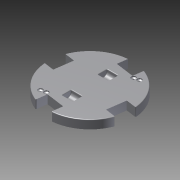
# Autodesk Inventor part: Outlet Cover [Top]
Saved by Autodesk Inventor 2012 (Build 160160000, 160)
## iProperties
Created: 2012-04-03
Part Number: Outlet Cover [Top]
Material: Default
Document SubType Name: Modeling
Designer: 21842
Density: 1 g/cm^3
Author: 21842
Autodesk Inventor part; units mm, degrees
ref_plane "YZ Plane" through (0, 0, 0) normal (1, 0, 0) x (0, 1, 0)
ref_plane "XZ Plane" through (0, 0, 0) normal (0, 1, 0) x (-1, 0, 0)
ref_plane "XY Plane" through (0, 0, 0) normal (0, 0, 1) x (1, 0, 0)
sketch "Sketch1" plane through (0, 0, 0) normal (0, 0, 1) x (1, 0, 0)
  circle A0 centre (-23.1688, -41.9) radius 3.5
  circle A1 centre (23.1688, 41.9) radius 3.5
  circle A2 centre (-30.3996, -43.4151) radius 3.5
  circle A3 centre (30.3996, 43.4151) radius 3.5
  circle A4 centre (-20.5794, 37.9797) radius 2.75
  circle A5 centre (20.5794, -37.9797) radius 2.75
  circle A6 centre (-30.3996, -43.4151) radius 1.6
  circle A7 centre (-23.1688, -41.9) radius 1.6
  circle A8 centre (23.1688, 41.9) radius 1.6
  circle A9 centre (30.3996, 43.4151) radius 1.6
  line L0 (-62.7781, -5.2832) -> (-47.4535, -7.4369)
  line L1 (-47.4535, -7.4369) -> (-43.6375, 19.715)
  line L2 (-43.6375, 19.715) -> (-59.0767, 21.8849)
  line L3 (5.2832, -62.7781) -> (7.4369, -47.4535)
  line L4 (7.4369, -47.4535) -> (-19.715, -43.6375)
  line L5 (-19.715, -43.6375) -> (-21.8849, -59.0767)
  line L6 (62.7781, 5.2832) -> (47.4535, 7.4369)
  line L7 (47.4535, 7.4369) -> (43.6375, -19.715)
  line L8 (43.6375, -19.715) -> (59.0767, -21.8849)
  line L9 (-5.2832, 62.7781) -> (-7.4369, 47.4535)
  line L10 (-7.4369, 47.4535) -> (19.715, 43.6375)
  line L11 (19.715, 43.6375) -> (21.8849, 59.0767)
  arc A10 (-5.2832, 62.7781) -> (-59.0767, 21.8849) centre (0, 0) ccw
  arc A11 (62.7781, 5.2832) -> (21.8849, 59.0767) centre (0, 0) ccw
  arc A12 (-62.7781, -5.2832) -> (-21.8849, -59.0767) centre (0, 0) ccw
  arc A13 (5.2832, -62.7781) -> (59.0767, -21.8849) centre (0, 0) ccw
  dimension "d0" = 3.2
  dimension "d1" = 3.2
  dimension "d2" = 3.2
  dimension "d3" = 3.2
  dimension "d8" = 360
  constraints: 24 end point, 14 centre point, 8 point on circle, 4 coincident, 29 other
  measures "d0" diameter of A6
  measures "d1" diameter of A7
  measures "d2" diameter of A8
  measures "d3" diameter of A9
extrude "Extrusion1" add sketch "Sketch1" along normal blind 12.7 contours A0 | A1 | A2 | A3 | A4 | A5 | L0 L1 L2 A10 L9 L10 L11 A11 L6 L7 L8 A13 L3 L4 L5 A12
extrude "Extrusion2" cut sketch "Sketch1" along normal blind 7 contours A4 | A5
hole "Hole1" at (30.3996, 43.4151, 12.7) direction (0, 0, -1) diameter 7 depth 1.5 tip angle 118
hole "Hole2" at (23.1688, 41.9, 12.7) direction (0, 0, -1) diameter 7 depth 1.5 tip angle 118
hole "Hole3" at (-23.1688, -41.9, 12.7) direction (0, 0, -1) diameter 7 depth 1.5 tip angle 118
hole "Hole4" at (-30.3996, -43.4151, 12.7) direction (0, 0, -1) diameter 7 depth 1.5 tip angle 118
extrude "Extrusion3" cut sketch "Sketch1" along normal blind 1.5 contours A2 | A3
sketch "Sketch3" plane through (0, 0, 0) normal (0, 0, -1) x (-1, 0, 0)
  arc A0 (21.8849, -59.0767) -> (62.7781, -5.2832) centre (0, 0) ccw projected
  line L0 (-15, 20) -> (-15, 40)
  line L1 (-15, 40) -> (15, 40)
  line L2 (15, -40) -> (-15, -40)
  line L3 (-15, -40) -> (-15, -20)
  line L4 (15, 40) -> (15, 20)
  line L5 (15, -20) -> (15, -40)
  arc A1 (-15, 20) -> (-15, -20) centre (0, 0) ccw
  arc A2 (15, -20) -> (15, 20) centre (0, 0) ccw
  constraints: 12 end point, 4 point on circle, 2 centre point, 2 perpendicular, 1 coincident, 1 parallel
extrude "Extrusion4" cut sketch "Sketch3" against normal blind 4
sketch "Sketch4" plane through (0, 0, 12.7) normal (0, 0, 1) x (1, 0, 0)
  line L0 (0, 20) -> (8, 20)
  line L1 (8, 20) -> (8, 33.4)
  line L2 (8, 33.4) -> (-8, 33.4)
  line L3 (-8, 33.4) -> (-8, 20)
  line L4 (-8, 20) -> (0, 20)
  line L5 (0, -20) -> (8, -20)
  line L6 (8, -20) -> (8, -33.4)
  line L7 (8, -33.4) -> (-8, -33.4)
  line L8 (-8, -33.4) -> (-8, -20)
  line L9 (-8, -20) -> (0, -20)
  arc A0 (-62.7781, -5.2832) -> (-21.8849, -59.0767) centre (0, 0) ccw projected
  arc A1 (5.2832, -62.7781) -> (59.0767, -21.8849) centre (0, 0) ccw projected
  dimension "d67" = 33.4
  dimension "d68" = 20
  dimension "d69" = 33.4
  dimension "d70" = 20
  constraints: 20 end point, 2 point on line, 1 collinear, 1 parallel, 1 perpendicular
  measures "d67" distance from line of A0.centre L2
  measures "d68" distance from line of A0.centre L4
  measures "d69" distance from line of L7 A1.centre
  measures "d70" distance from line of A0.centre L9
extrude "Extrusion5" cut sketch "Sketch4" against normal blind 8
fillet "Fillet1" radius 1 12 edges at (-50.1537, -38.1263, 12.7) (-38.1263, 50.1537, 12.7) (50.1537, 38.1263, 12.7) (38.1263, -50.1537, 12.7) (-21.8849, -59.0767, 6.35) (5.2832, -62.7781, 6.35) (59.0767, -21.8849, 6.35) (62.7781, 5.2832, 6.35) (21.8849, 59.0767, 6.35) (-5.2832, 62.7781, 6.35) (-59.0767, 21.8849, 6.35) (-62.7781, -5.2832, 6.35)
fillet "Fillet2" radius 5 4 edges at (0, -20, 4.7) (0, 20, 4.7) (0, -33.4, 4.7) (0, 33.4, 4.7)
fillet "Fillet3" radius 1 28 edges at (0, -20, 12.7) (8, -26.7, 12.7) (0, -33.4, 12.7) (-8, -26.7, 12.7) (-8, 26.7, 12.7) (0, 33.4, 12.7) (8, 26.7, 12.7) (0, 20, 12.7) (-8, 33.4, 11.2) (-8, 26.7, 4.7) (-8, 21.4645, 6.1645) (-8, 20, 11.2) (-8, 31.9355, 6.1645) (8, 21.4645, 6.1645) (8, 26.7, 4.7) (8, 31.9355, 6.1645) (8, 33.4, 11.2) (8, 20, 11.2) (8, -26.7, 4.7) (8, -31.9355, 6.1645) (8, -33.4, 11.2) (8, -20, 11.2) (8, -21.4645, 6.1645) (-8, -21.4645, 6.1645) (-8, -26.7, 4.7) (-8, -31.9355, 6.1645) (-8, -33.4, 11.2) (-8, -20, 11.2)
body "Solid1"
